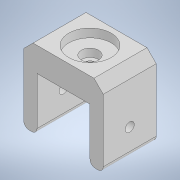
# Autodesk Inventor part: Magnet Mount
Saved by Autodesk Inventor 2022 (Build 260153000, 153)
## iProperties
Created: 2022-03-20
Part Number: Magnet Mount
Material: Generic
Document SubType Name: Modeling
Designer: Nick
Density: 1 g/cm^3
Appearance: Default
Author: Nick
Autodesk Inventor part; units mm, degrees
ref_plane "YZ Plane" through (0, 0, 0) normal (1, 0, 0) x (0, 1, 0)
ref_plane "XZ Plane" through (0, 0, 0) normal (0, 1, 0) x (-1, 0, 0)
ref_plane "XY Plane" through (0, 0, 0) normal (0, 0, 1) x (1, 0, 0)
sketch "Sketch1" plane through (0, 0, 0) normal (0, 1, 0) x (-1, 0, 0)
  circle A0 centre (0, 0) radius 8
  line L0 (15, -10) -> (-15, -10)
  line L1 (-15, -10) -> (-15, 10)
  line L2 (-15, 10) -> (15, 10)
  line L3 (15, 10) -> (15, -10)
  point P0 (-15, 0)
  point P1 (0, -10)
  dimension "d0" = 30
  dimension "d1" = 16
  dimension "d2" = 20
  constraints: 8 end point, 2 midpoint, 2 parallel, 1 centre point, 1 coincident, 1 horizontal, 1 horizontal alignment, 1 perpendicular, 1 vertical alignment
  measures "d0" distance of L0.start L0.end
  measures "d1" diameter of A0
  measures "d2" distance of L0.end L1.end
extrude "Extrusion1" add sketch "Sketch1" against normal blind 6 contours A0 | L0 L1 L2 L3
extrude "Extrusion2" add sketch "Sketch1" along normal blind 3.2
hole "Hole1" at (0, 0, 0) direction (0, -1, 0) diameter 3.4 depth 10 counterbore diameter 6.5 counterbore depth 3.05 clearance for "Socket Head Cap Screw" size "M3" standard "Ansi Metric M Profile"
sketch "Sketch2" plane through (0, -6, 0) normal (0, -1, 0) x (1, 0, 0)
  circle A0 centre (0, 0) radius 1.7 projected
  line L0 (15, 10) -> (-15, 10) projected
  line L1 (-15, 10) -> (-15, -10) projected
  line L2 (-15, -10) -> (15, -10) projected
  line L3 (15, -10) -> (15, 10) projected
  line L4 (-15, 10) -> (-15, -10) projected
  line L5 (-15, 10) -> (-10, 10)
  line L6 (-10, 10) -> (-10, -10)
  line L7 (-10, -10) -> (-15, -10)
  line L8 (-15, -10) -> (-15, 10)
  line L9 (-15, -10) -> (15, -10) projected
  line L10 (15, 10) -> (-15, 10) projected
  line L11 (15, -10) -> (10, -10)
  line L12 (10, -10) -> (10, 10)
  line L13 (10, 10) -> (15, 10)
  line L14 (15, 10) -> (15, -10)
  point P0 (10, 10)
  dimension "d14" = 5
  dimension "d15" = 5
  constraints: 16 end point, 4 parallel, 2 horizontal, 2 perpendicular, 2 point on line
  measures "d14" distance between parallel lines of L3 L12
  measures "d15" distance between parallel lines of L1 L6
extrude "Extrusion3" add sketch "Sketch2" along normal blind 20 contours L3 L2 L12 L0 | L6 L2 L1 L0
chamfer "Chamfer1" distance 3.5 angle 45 2 edges at (15, 3.2, 0) (-15, 3.2, 0)
fillet "Fillet1" radius 2 4 edges at (-15, -26, 0) (-10, -26, 0) (10, -26, 0) (15, -26, 0)
sketch "Sketch3" plane through (15, -0.3, 10) normal (1, 0, 0) x (0, 0, -1)
  line L0 (20, -23.7) -> (0, -23.7) projected
  line L1 (20, -5.7) -> (20, -23.7) projected
  line L2 (0, -5.7) -> (20, -5.7) projected
  line L3 (0, -5.7) -> (0, -23.7) projected
  line L4 (0, -25.7) -> (20, -25.7) projected
  line L5 (20, -25.7) -> (0, -25.7) projected
  line L6 (0, -5.7) -> (0, -23.7) projected
  line L7 (0, -25.7) -> (0, -5.7)
  point P0 (10, 0.3)
  point P1 (0, -15.7)
  point P2 (10, -25.7)
  point P3 (10, -25.7)
  point P4 (10, -15.7)
  constraints: 3 midpoint, 2 end point, 1 collinear, 1 horizontal alignment, 1 vertical alignment
hole "Hole2" at (15, -16, 0) direction (-1, 0, 0) diameter 3.4 end through all
equation "\"d15\" = d14"
body "Solid1"
